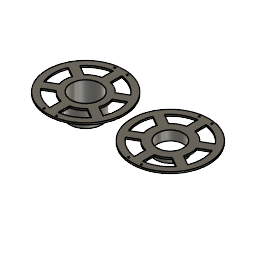
MiniSpool (Autodesk Fusion 360 design; units mm, degrees)
Autodesk Fusion 360 part; units mm, degrees
note: some values were not read from the file. Set by a fixed rule: which sketch regions a step uses.
sketch "Sketch1" plane through (0, 0, 0) normal (0, 0, 1) x (1, 0, 0)
  circle A0 centre (0, 0) radius 72.5
  circle A1 centre (0, 0) radius 27.5
  circle A2 centre (0, 0) radius 30.5
  circle A3 centre (0, 0) radius 60.5
  circle A4 centre (0, 0) radius 39.5
  line L0 (0, 74) -> (0, 30.5)
  line L1 (8, 72.0573) -> (8, 38.6814)
  line L2 (-8, 72.0573) -> (-8, 38.6814)
  line L3 (-66.4034, 29.1004) -> (-37.4991, 12.4125)
  line L4 (-58.4034, 42.9568) -> (-29.4991, 26.2689)
  line L5 (-58.4034, -42.9568) -> (-29.4991, -26.2689)
  line L6 (-66.4034, -29.1004) -> (-37.4991, -12.4125)
  line L7 (8, -72.0573) -> (8, -38.6814)
  line L8 (-8, -72.0573) -> (-8, -38.6814)
  line L9 (66.4034, -29.1004) -> (37.4991, -12.4125)
  line L10 (58.4034, -42.9568) -> (29.4991, -26.2689)
  line L11 (58.4034, 42.9568) -> (29.4991, 26.2689)
  line L12 (66.4034, 29.1004) -> (37.4991, 12.4125)
  circle A5 centre (0, 0) radius 68
  circle A6 centre (-12, 66.9328) radius 1.5
  circle A7 centre (12, 66.9328) radius 1.5
  circle A8 centre (12, -66.9328) radius 1.5
  circle A9 centre (-12, -66.9328) radius 1.5
  dimension "d1" = 145
  dimension "d2" = 55
  dimension "d3" = 61
  dimension "d4" = 121
  dimension "d5" = 79
  dimension "d6" = 8
  dimension "d7" = 8
  dimension "d9" = 360
  dimension "d10" = 136
  dimension "d11" = 3
  dimension "d12" = 3
  dimension "d13" = 4
  dimension "d14" = 4
  dimension "d16" = 360
  constraint coincident A0.centre A1.centre
  constraint concentric A0 A1
  constraint concentric A2 A4
  constraint coincident A2 L0.end
  constraint vertical L0
  constraint coincident A0 L1.start
  constraint coincident A4 L1.end
  constraint parallel L0 L1
  constraint coincident A0 L2.start
  constraint coincident A4 L2.end
  constraint parallel L1 L2
  constraint concentric A4 A5
  constraint coincident A5 A6.centre
  constraint coincident A5 A7.centre
  measures "d1" diameter of A0
  measures "d2" diameter of A1
  measures "d3" diameter of A2
  measures "d4" diameter of A3
  measures "d5" diameter of A4
  measures "d6" distance of L0 L2
  measures "d7" distance of L0 L1
  measures "d10" diameter of A5
  measures "d11" diameter of A6
  measures "d12" diameter of A7
  measures "d13" distance of L2 A6.centre
  measures "d14" distance of L1 A7.centre
extrude "Extrude1" add sketch "Sketch1" along normal blind 3 contours A0 L9 L12 A5 | A0 L11 L12 A5 | A0 L9 L10 A5 | A0 L1 L11 A5 A7 | A3 L9 L12 A5 | A3 L11 L12 A5 | A0 L7 L10 A5 A8 | A3 L9 L10 A5 | A0 L0 L1 A5 | A3 L1 L11 A5 A7 | A3 A4 L11 L12 | A0 L7 L8 A5 | A3 L7 L10 A5 A8 | A3 A4 L9 L10 | A0 L0 L2 A5 | A3 L0 L1 A5 | A4 | A0 L5 L8 A5 A9 | A3 L7 L8 A5 | A0 L2 L4 A5 A6 | A3 L0 L2 A5 | A3 A4 L0 L1 | A0 L5 L6 A5 | A3 L5 L8 A5 A9 | A3 A4 L7 L8 | A0 L3 L4 A5 | A3 L2 L4 A5 A6 | A3 A4 L0 L2 | A0 L3 L6 A5 | A3 L5 L6 A5 | A3 L3 L4 A5 | A3 L3 L6 A5 | A3 A4 L5 L6 | A3 A4 L3 L4 | A2 makes body 1
extrude "Extrude2" add sketch "Sketch1" against normal blind 36 contours A2 bodies 1
sketch "Sketch2" plane through (0, 0, 0) normal (0, 0, 1) x (1, 0, 0)
  circle A0 centre (160, 0) radius 68
  circle A1 centre (160, 0) radius 72.5
  circle A2 centre (148, -66.9328) radius 1.5
  line L0 (168, -72.0573) -> (168, -38.6814)
  line L1 (226.4034, -29.1004) -> (197.4991, -12.4125)
  line L2 (168, 72.0573) -> (168, 38.6814)
  line L3 (101.5966, 42.9568) -> (130.5009, 26.2689)
  line L4 (101.5966, -42.9568) -> (130.5009, -26.2689)
  circle A3 centre (172, -66.9328) radius 1.5
  line L5 (93.5966, 29.1004) -> (122.5009, 12.4125)
  circle A4 centre (148, 66.9328) radius 1.5
  line L6 (218.4034, 42.9568) -> (189.4991, 26.2689)
  line L7 (93.5966, -29.1004) -> (122.5009, -12.4125)
  circle A5 centre (160, 0) radius 39.5
  line L8 (218.4034, -42.9568) -> (189.4991, -26.2689)
  circle A6 centre (172, 66.9328) radius 1.5
  circle A7 centre (160, 0) radius 30.5
  line L9 (152, -72.0573) -> (152, -38.6814)
  circle A8 centre (160, 0) radius 60.5
  line L10 (152, 72.0573) -> (152, 38.6814)
  circle A9 centre (160, 0) radius 27.5
  line L11 (226.4034, 29.1004) -> (197.4991, 12.4125)
  line L12 (160, 74) -> (160, 30.5)
  circle A10 centre (160, 0) radius 24.5
  point P0 (160, 0)
  dimension "d23" = 360
  dimension "d25" = 360
  dimension "d26" = 145
  dimension "d27" = 55
  dimension "d28" = 61
  dimension "d29" = 121
  dimension "d30" = 79
  dimension "d31" = 8
  dimension "d32" = 8
  dimension "d33" = 136
  dimension "d34" = 3
  dimension "d35" = 3
  dimension "d36" = 4
  dimension "d37" = 4
  dimension "d38" = 49
  constraint coincident P0 A0.centre
  constraint concentric A1 A9
  constraint concentric A5 A7
  constraint coincident L12.end A7
  constraint vertical L12
  constraint coincident L2.start A1
  constraint coincident L2.end A5
  constraint parallel L2 L12
  constraint coincident L10.start A1
  constraint coincident L10.end A5
  constraint parallel L2 L10
  constraint concentric A0 A5
  constraint coincident A4.centre A0
  constraint coincident A6.centre A0
  constraint concentric A8 A10
  measures "d26" diameter of A1
  measures "d27" diameter of A9
  measures "d28" diameter of A7
  measures "d29" diameter of A8
  measures "d30" diameter of A5
  measures "d31" distance of L10 L12
  measures "d32" distance of L2 L12
  measures "d33" diameter of A0
  measures "d34" diameter of A4
  measures "d35" diameter of A6
  measures "d36" distance of A4.centre L10
  measures "d37" distance of A6.centre L2
  measures "d38" diameter of A10
extrude "Extrude3" add sketch "Sketch2" along normal blind 3 separate body contours A0 L1 A8 L11 | A0 A1 L1 L11 | A0 L6 A8 L11 | A0 A1 L6 L11 | A0 A1 L1 L8 | A0 L1 L8 A8 | A0 L2 L6 A6 A8 | A0 A1 L2 L6 A6 | L6 A5 A8 L11 | A0 A1 L0 A3 L8 | A0 L0 A3 L8 A8 | L1 A5 L8 A8 | A5 | A0 A1 L2 L12 | A0 L2 A8 L12 | L2 A5 A8 L12 | A0 A1 L0 L9 | L0 A5 L9 A8 | A0 L0 L9 A8 | A0 A1 L10 L12 | A5 A8 L10 L12 | A0 A8 L10 L12 | A0 A1 A2 L4 L9 | A0 A2 L4 L9 A8 | A0 A1 L3 A4 L10 | A0 L3 A4 A8 L10 | A0 A1 L4 L7 | L4 L7 A5 A8 | A0 L4 L7 A8 | A0 A1 L3 L5 | A0 L3 L5 A8 | L3 L5 A5 A8 | A0 A1 L5 L7 | A0 L5 L7 A8 | A7 | A9 makes body 2
extrude "Extrude4" add sketch "Sketch2" against normal blind 15 contours A9 bodies 2
